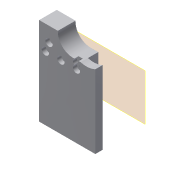
# Autodesk Inventor part: cellSTORM_cellphone_plate
Saved by Autodesk Inventor 2019 (Build 230136000, 136)
## iProperties
Created: 2020-02-11
Part Number: cellSTORM_cellphone_plate
Material: Generic
Document SubType Name: Modeling
Designer: diederichbenedict
Density: 1 g/cm^3
Appearance: White
Author: diederichbenedict
Autodesk Inventor part; units mm, degrees
ref_plane "YZ Plane" through (0, 0, 0) normal (1, 0, 0) x (0, 1, 0)
ref_plane "XZ Plane" through (0, 0, 0) normal (0, 1, 0) x (-1, 0, 0)
ref_plane "XY Plane" through (0, 0, 0) normal (0, 0, 1) x (1, 0, 0)
ref_plane "Work Plane2" through (4.5, -13.125, 5) normal (0, 0, 1) x (1, 0, 0)
sketch "Sketch5" plane through (4.5, -13.125, 5) normal (0, 0, 1) x (1, 0, 0)
  circle A0 centre (-5.3843, -10.9183) radius 3.5 projected
  line L0 (40.5, 19.8795) -> (20.6391, 19.8795) projected
  line L1 (20.6391, 19.8795) -> (-0.5, 15.425) projected
  line L2 (-0.5, 15.425) -> (-8.5, 15.425) projected
  line L3 (-8.5, 15.425) -> (-8.5, 12.625) projected
  line L4 (-8.5, 12.625) -> (-22.6946, 12.625) projected
  line L5 (-22.6946, 12.625) -> (-28.1392, 19.0495) projected
  arc A1 (-28.1392, 19.0495) -> (-34.556, 17.8156) centre (-31, 16.625) ccw projected
  spline S0 degree 3 poles (-34.556, 17.8156) (-34.7591, 16.8991) (-35.0888, 16.002) (-36.0242, 14.6392) (-36.5194, 14.1543) (-37.6005, 13.4479) (-38.1283, 13.21) (-39.2688, 12.8371) (-39.8866, 12.7101) (-40.5, 12.625) knots 0 0 0 0 0.281642 0.281642 0.494296 0.494296 0.667567 0.667567 0.853113 0.853113 0.853113 0.853113 projected
  line L6 (-40.5, 12.625) -> (-40.5, 2.625) projected
  line L7 (-40.5, 2.625) -> (-0.5, 2.625) projected
  line L8 (-0.5, 2.625) -> (20.6391, 7.0795) projected
  line L9 (20.6391, 7.0795) -> (20.6391, -0.375) projected
  line L10 (20.6391, -0.375) -> (-19.5, -0.375) projected
  line L11 (-19.5, -0.375) -> (-19.5, -6.375) projected
  line L12 (-19.5, -6.375) -> (-16.1781, -6.375) projected
  line L13 (-16.1781, -6.375) -> (-16.1781, -20.375) projected
  line L14 (-16.1781, -20.375) -> (5.3645, -20.375) projected
  line L15 (5.3645, -20.375) -> (5.3645, -6.375) projected
  line L16 (5.3645, -6.375) -> (40.5, -6.375) projected
  line L17 (40.5, -6.375) -> (40.5, 19.8795) projected
  line L18 (20.6391, 19.3686) -> (20.6391, 7.5905) projected
  line L19 (20.6391, 7.5905) -> (17.9999, 7.0344) projected
  line L20 (17.9999, 7.0344) -> (17.2782, 10.4592) projected
  line L21 (17.2782, 10.4592) -> (2.6006, 7.3662) projected
  line L22 (2.6006, 7.3662) -> (3.3222, 3.9414) projected
  line L23 (3.3222, 3.9414) -> (-0.5, 3.136) projected
  line L24 (-0.5, 3.136) -> (-0.5, 14.914) projected
  line L25 (-0.5, 14.914) -> (2.9614, 15.6434) projected
  line L26 (2.9614, 15.6434) -> (3.6831, 12.2186) projected
  line L27 (3.6831, 12.2186) -> (18.3608, 15.3116) projected
  line L28 (18.3608, 15.3116) -> (17.6391, 18.7364) projected
  line L29 (17.6391, 18.7364) -> (20.6391, 19.3686) projected
  circle A2 centre (-4.5, 7.625) radius 1.4 projected
  circle A3 centre (-4.5, 12.625) radius 1.4 projected
  circle A4 centre (-19.5, 7.625) radius 1.4 projected
  circle A5 centre (-34.5, 7.625) radius 1.4 projected
  circle A6 centre (-31, 16.625) radius 1.5 projected
  line L30 (-0.5, 2.625) -> (-0.5, 15.425)
  line L31 (-22.6946, 12.625) -> (-40.5, 12.625)
  arc A7 (-22.5, 30.625) -> (-8.5, 15.425) centre (-8.0073, 29.9262) ccw projected
  line L32 (-22.5, 30.625) -> (-40.5, 30.625) projected
  line L33 (-40.5, 30.625) -> (-40.5, 2.625) projected
  circle A8 centre (-31, 27.1712) radius 1.4 projected
  point P0 (-4.5, 13.125)
  constraints: 4 end point, 1 collinear, 1 horizontal
extrude "Extrusion3" add sketch "Sketch5" along normal blind 10 contours L30 L24 L7 L6 L31 L4 L3 L2 | L3 L4 L5 A1 S0 L33 L32 A7 | L31 S0 A1 L5
sketch "Sketch6" plane through (4.5, -13.125, 15) normal (0, 0, 1) x (1, 0, 0)
  circle A0 centre (-34.5, 7.625) radius 1.4 projected
  circle A1 centre (-19.5, 7.625) radius 1.4 projected
  circle A2 centre (-4.5, 12.625) radius 1.4 projected
  circle A3 centre (-4.5, 7.625) radius 1.4 projected
  line L0 (-0.5, 15.425) -> (-8.5, 15.425) projected
  line L1 (-40.5, 30.625) -> (-40.5, 2.625) projected
  line L2 (-40.5, 2.625) -> (-0.5, 2.625) projected
  line L3 (-0.5, 2.625) -> (-0.5, 15.425) projected
  circle A4 centre (4.9975, 34.5751) radius 13.9 construction
  line L4 (-0.5, 2.625) -> (-0.5, 15.425) projected
  arc A5 (-0.5, 15.425) -> (13.6114, 16.6099) centre (4.9975, 34.5751) ccw
  line L5 (-8.5, 12.625) -> (-40.5, 12.625) projected
  line L6 (-40.5, 12.625) -> (-40.5, 34.5751)
  line L7 (-40.5, 34.5751) -> (-14.9261, 34.5751)
  line L8 (13.6114, 16.6099) -> (13.6114, -54.1295)
  line L9 (13.6114, 16.6099) -> (84.3508, 16.6099) construction
  line L10 (13.6114, -54.1295) -> (-40.5, -54.1295)
  line L11 (-40.5, -54.1295) -> (-40.5, 2.625)
  arc A6 (-22.5, 30.625) -> (-8.5, 15.425) centre (-8.0073, 29.9262) ccw projected
  line L12 (-22.5, 30.625) -> (-40.5, 30.625) projected
  circle A7 centre (-8.0073, 29.9262) radius 14.5095
  line L13 (-40.5, 30.625) -> (-40.5, 2.625) projected
  line L14 (-40.5, 30.625) -> (-40.5, 40.6638)
  line L15 (-8.0073, 44.4357) -> (-8.0073, 46.4357)
  line L16 (-8.0073, 46.4357) -> (-40.5, 46.4357)
  line L17 (-40.5, 46.4357) -> (-40.5, 30.625)
  line L18 (-22.5, 30.625) -> (-40.5, 30.625) projected
  line L19 (-22.5, 30.625) -> (-40.5, 30.625)
  point P0 (-4.5, 13.125)
  dimension "d15" = 90
  dimension "d25" = 2
  dimension "d26" = 90
  constraints: 23 end point, 4 perpendicular, 3 vertical, 2 coincident, 2 horizontal, 2 point on circle, 1 centre point, 1 collinear, 1 vertical alignment, 2 other
  measures "d15" angle of L8 L9
  measures "d25" distance of L15.start L15.end
  measures "d26" angle of L16 L15
extrude "Extrusion4" add sketch "Sketch6" along normal blind 7 contours L3 L2 L1 L12 A6 A7 L0 | A5 L8 L10 L11 L2 L3 | A7 L0
sketch "Sketch7" plane through (4.5, -13.125, 22) normal (0, 0, 1) x (1, 0, 0)
  circle A0 centre (-19.5, 7.625) radius 1.4 projected
  circle A1 centre (-34.5, 7.625) radius 1.4 projected
  circle A2 centre (-4.5, 7.625) radius 1.4 projected
  circle A3 centre (-4.5, 12.625) radius 1.4 projected
  circle A4 centre (-31, 16.625) radius 1.5 projected
  circle A5 centre (-4.5, 7.625) radius 1.4 projected
  circle A6 centre (-4.5, 12.625) radius 1.4 projected
  circle A7 centre (-19.5, 7.625) radius 1.4 projected
  circle A8 centre (-34.5, 7.625) radius 1.4 projected
  line L0 (-0.5, 15.425) -> (-8.5, 15.425) projected
  arc A9 (-22.5, 30.625) -> (-8.5, 15.425) centre (-8.0073, 29.9262) ccw projected
  line L1 (-22.5, 30.625) -> (-40.5, 30.625) projected
  line L2 (-40.5, 30.625) -> (-40.5, -54.1295) projected
  line L3 (-40.5, -54.1295) -> (13.6114, -54.1295) projected
  line L4 (13.6114, -54.1295) -> (13.6114, 16.6099) projected
  arc A10 (-0.5, 15.425) -> (13.6114, 16.6099) centre (4.9975, 34.5751) ccw projected
  circle A11 centre (-31, 27.1712) radius 1.4 projected
  circle A12 centre (-7, -33.875) radius 1.95 projected
  point P0 (-4.5, 13.125)
hole "Hole2" at (-30, -5.5, 22) at (-15, -5.5, 22) at (0, -5.5, 22) at (0, -0.5, 22) at (-26.5, 3.5, 22) at (-2.5, -47, 22) at (-26.5, 14.0462, 22) direction (0, 0, -1) diameter 2.9 end through all counterbore diameter 7 counterbore depth 4
body "Solid2"
